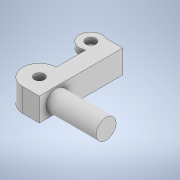
# Autodesk Inventor part: stuur_ARMPJE
Saved by Autodesk Inventor 2022 (Build 260153000, 153)
## iProperties
Created: 2021-11-25
Part Number: stuur_ARMPJE
Material: Generic
Document SubType Name: Modeling
Designer: keemi
Density: 1 g/cm^3
Appearance: Default
Author: keemi
Autodesk Inventor part; units mm, degrees
ref_plane "YZ Plane" through (0, 0, 0) normal (1, 0, 0) x (0, 1, 0)
ref_plane "XZ Plane" through (0, 0, 0) normal (0, 1, 0) x (-1, 0, 0)
ref_plane "XY Plane" through (0, 0, 0) normal (0, 0, 1) x (1, 0, 0)
sketch "Sketch1" plane through (0, 0, 0) normal (0, 1, 0) x (-1, 0, 0)
  circle A0 centre (0, 0) radius 1.5
  circle A1 centre (0, 0) radius 5
  line L0 (-5, 0) -> (-5, 5)
  line L1 (-5, 5) -> (0, 5)
  line L2 (-5, 0) -> (-5, -20)
  line L3 (-5, -20) -> (-1.5, -20)
  line L4 (-5, -20) -> (0, -20)
  line L5 (0, -20) -> (0, -5)
  dimension "d0" = 3
  dimension "d1" = 10
  dimension "d2" = 20
  constraints: 12 end point, 3 point on circle, 2 centre point, 2 coincident, 2 perpendicular, 2 point on line, 2 tangent, 1 vertical
  measures "d0" diameter of A0
  measures "d1" diameter of A1
  measures "d2" distance of L0.start L2.end
extrude "Extrusion1" add sketch "Sketch1" along normal blind 7
sketch "Sketch2" plane through (5, 0, 5) normal (1, 0, 0) x (0, 0, -1)
  line L0 (10, 7) -> (0, 7) projected
  line L1 (0, 7) -> (0, 3.5)
  line L2 (0, 0) -> (25, 0) projected
  line L3 (0, 3.5) -> (5, 3.5)
  circle A0 centre (5, 3.5) radius 3
  point P0 (5, 0)
  dimension "d5" = 3.5
  dimension "d6" = 6
  constraints: 4 end point, 2 perpendicular, 1 centre point, 1 coincident
  measures "d5" distance of L0.end L1.end
  measures "d6" diameter of A0
extrude "Extrusion2" add sketch "Sketch2" along normal blind 15
sketch "Sketch3" plane through (5, 0, 5) normal (1, 0, 0) x (0, 0, -1)
  point P0 (5, 0)
sketch "Sketch7" plane through (0, 7, 0) normal (0, 1, 0) x (1, 0, 0)
  line L0 (0, 19.9362) -> (0, 16.9362)
  line L1 (0, 20) -> (0, 5) projected
  line L2 (0, 16.9362) -> (-1.5, 16.9362)
  circle A0 centre (-1.5, 16.9362) radius 1.5
  circle A1 centre (-1.5, 16.9362) radius 3.4113
  point P0 (0, 0)
  point P1 (0, 13.8723)
  dimension "d25" = 3
  dimension "d26" = 1.5
  constraints: 4 end point, 2 coincident, 1 horizontal, 1 horizontal alignment, 1 point on line, 5 other
  measures "d25" distance of L0.start L0.end
  measures "d26" distance of L0.end L2.end
extrude "Extrusion6" add sketch "Sketch7" against normal blind 7 contours L0 L1 A1 picked at (-0.578, 19.5142)
sketch "Sketch8" plane through (0, 0, -5) normal (-1, 0, 0) x (0, 0, 1)
  line L0 (-8.8723, 7) -> (0, 7) projected
  line L1 (-7.6834, 7) -> (-4.1834, 7)
  line L2 (-7.6834, 7) -> (-7.6834, 3.5)
  line L3 (-7.6834, 7) -> (-4.1834, 7) construction
  line L4 (-7.6834, 3.5) -> (-7.6834, 1.8)
  line L5 (-7.6834, 1.8) -> (-17.6834, 1.8)
  line L6 (-17.6834, 1.8) -> (-17.6834, 5.2)
  line L7 (-17.6834, 5.2) -> (-7.6834, 5.2)
  line L8 (-7.6834, 5.2) -> (-7.6834, 1.8)
  point P0 (5, 0)
  point P1 (-7.6834, 5.2)
  dimension "d29" = 3.5
  dimension "d30" = 3.5
  dimension "d31" = 90
  dimension "d32" = 1.7
  dimension "d33" = 10
  dimension "d34" = 3.4
  constraints: 16 end point, 3 perpendicular, 3 point on line, 2 horizontal, 2 parallel
  measures "d29" distance of L1.start L1.end
  measures "d30" distance of L1.start L2.end
  measures "d31" angle of L2 L3
  measures "d32" distance of L2.end L4.end
  measures "d33" distance of L6.end L7.end
  measures "d34" distance of L5.end L6.end
extrude "Extrusion7" cut sketch "Sketch8" along normal blind 7
body "Solid1"
